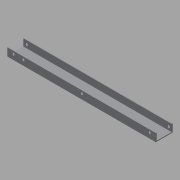
# Autodesk Inventor part: 26in C-Channel (TopPlate Supports)
Saved by Autodesk Inventor 2013 (Build 170138000, 138)
## iProperties
Created: 2013-01-27
Part Number: 26in C-Channel (TopPlate Supports)
Material: Aluminum 6061
Document SubType Name: Modeling
Designer: Naphat
Density: 1 g/cm^3
Author: Naphat
Autodesk Inventor part; units mm, degrees
ref_plane "YZ Plane" through (0, 0, 0) normal (1, 0, 0) x (0, 1, 0)
ref_plane "XZ Plane" through (0, 0, 0) normal (0, 1, 0) x (-1, 0, 0)
ref_plane "XY Plane" through (0, 0, 0) normal (0, 0, 1) x (1, 0, 0)
sketch "Sketch1" plane through (0, 0, 0) normal (1, 0, 0) x (0, 1, 0)
  line L0 (0, 0) -> (0, -40)
  line L1 (0, -40) -> (19, -40)
  line L2 (19, -40) -> (19, -38)
  line L3 (0, 0) -> (19, 0)
  line L4 (19, 0) -> (19, -2)
  line L5 (0, -20) -> (2, -20) construction
  line L6 (19, -2) -> (2, -2)
  line L7 (2, -2) -> (2, -38)
  line L8 (2, -38) -> (19, -38)
  dimension "d0" = 40
  dimension "d1" = 19
  dimension "d2" = 2
  dimension "d3" = 2
  dimension "d4" = 2
  constraints: 18 end point, 6 perpendicular, 2 parallel, 1 midpoint, 1 vertical
  measures "d0" distance of L0.start L0.end
  measures "d1" distance of L0.end L1.end
  measures "d2" distance of L1.end L2.end
  measures "d3" distance of L3.end L4.end
  measures "d4" distance of L5.start L5.end
extrude "Extrusion1" add sketch "Sketch1" along normal blind 355.6
sketch "Sketch2" plane through (0, 2, -2) normal (0, 0, -1) x (-1, 0, 0)
  circle A0 centre (-13.8784, 10.3) radius 3.175
  point P0 (0, -2)
  constraints: 1 centre point
extrude "Extrusion2" cut sketch "Sketch2" against normal blind 25.4
sketch "Sketch3" plane through (0, 2, -2) normal (0, 0, -1) x (-1, 0, 0)
  circle A0 centre (-13.8784, 10.3) radius 3.175
  line L0 (-355.6, 0) -> (-355.6, 17)
  line L1 (0, 17) -> (-355.6, 17)
  circle A1 centre (-37.4708, 10.3) radius 3.175
  circle A2 centre (-177.8, 10.3) radius 3.175
  circle A3 centre (-340.3166, 10.3) radius 3.175
  point P0 (0, -2)
  dimension "d9" = 6.35
  dimension "d10" = 6.35
  dimension "d11" = 6.35
  constraints: 4 centre point, 4 end point
  measures "d9" diameter of A1
  measures "d10" diameter of A2
  measures "d11" diameter of A3
extrude "Extrusion3" cut sketch "Sketch3" against normal blind 25.4 contours A1 | A2 | A3
sketch "Sketch4" plane through (0, 0, -40) normal (0, 0, -1) x (-1, 0, 0)
  circle A0 centre (-348.1, 9.62) radius 3.175
  circle A1 centre (-7.5, 9.62) radius 3.175
  constraints: 2 centre point
extrude "Extrusion4" cut sketch "Sketch4" against normal blind 25.4
body "Solid1"
